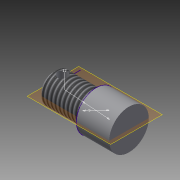
# Autodesk Inventor part: Tengely
Saved by Autodesk Inventor 2015 (Build 190159000, 159)
## iProperties
Created: 2014-09-27
Part Number: Tengely
Material: Generic
Document SubType Name: Modeling
Designer: laca
Density: 1 g/cm^3
Appearance: Default
Mass: 1.88179 g
Surface Area: 10.2081 cm^2
Volume: 1.88179 cm^3
Author: laca
Autodesk Inventor part; units mm, degrees
ref_plane "YZ Plane" through (0, 0, 0) normal (1, 0, 0) x (0, 1, 0)
ref_plane "XZ Plane" through (0, 0, 0) normal (0, 1, 0) x (-1, 0, 0)
ref_plane "XY Plane" through (0, 0, 0) normal (0, 0, 1) x (1, 0, 0)
sketch "Sketch1" plane through (0, 0, 0) normal (1, 0, 0) x (0, 1, 0)
  circle A0 centre (0, 0) radius 6
  circle A1 centre (0, 0) radius 4.5
  dimension "d0" = 12
  dimension "d1" = 9
  constraints: 2 centre point, 2 coincident
  measures "d0" diameter of A0
  measures "d1" diameter of A1
extrude "Extrusion1" add sketch "Sketch1" along normal blind 10 contours A0 | A1
extrude "Extrusion2" add sketch "Sketch1" against normal blind 13 contours A1
chamfer "Chamfer1" distance 1 angle 45 1 edges at (-13, -4.5, 0)
thread "Thread1" size "M9x1.25" class "6g" standard "ANSI Metric M Profile" full length
sketch "Sketch2" plane through (-13, 0, 0) normal (-1, 0, 0) x (0, 0, 1)
  line L0 (0, 0) -> (-8.2207, 0)
  constraints: 2 end point, 1 horizontal
ref_plane "Work Plane1" through (-13, 0, 0) normal (0, 1, 0) x (0, 0, -1)
sketch "Sketch3" plane through (-13, 0, 0) normal (0, 1, 0) x (0, 0, -1)
  circle A0 centre (0, -3) radius 1.5
  line L0 (6, -13) -> (-6, -13) projected
  point P0 (0, -13)
  dimension "d12" = 3
  dimension "d13" = 10
  constraints: 1 centre point
  measures "d12" diameter of A0
  measures "d13" distance from line of L0 A0.centre
extrude "Extrusion3" cut sketch "Sketch3" along normal blind 10 and the other way blind 5
body "Solid1"
